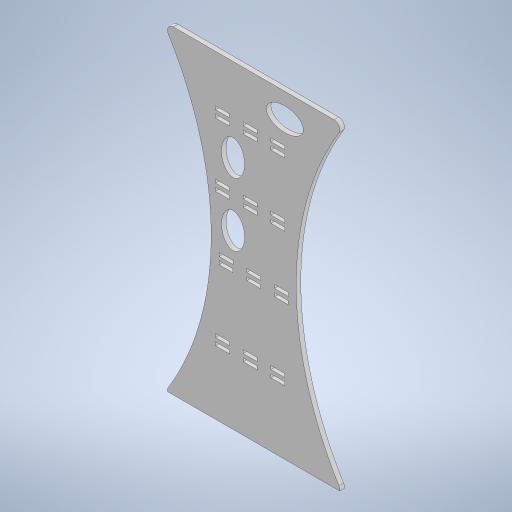
# Autodesk Inventor part: ребро
Saved by Autodesk Inventor 2023.1 (Build 271208000, 208)
## iProperties
Created: 2025-01-17
Part Number: ребро
Material: Типовые
Document SubType Name: Modeling
Designer: Коноваленко
Density: 1 g/cm^3
Appearance: По умолчанию
Author: Коноваленко
Autodesk Inventor part; units mm, degrees
ref_plane "YZ Plane" through (0, 0, 0) normal (1, 0, 0) x (0, 1, 0)
ref_plane "XZ Plane" through (0, 0, 0) normal (0, 1, 0) x (-1, 0, 0)
ref_plane "XY Plane" through (0, 0, 0) normal (0, 0, 1) x (1, 0, 0)
sketch "Эскиз1" plane through (0, 0, 0) normal (0, 0, 1) x (1, 0, 0)
  line L0 (81.8324, 0) -> (81.8324, -4) construction
  line L1 (72.759, -4) -> (11.9953, -4)
  line L2 (11.9953, -4) -> (11.9953, 0) construction
  line L3 (11.9953, 0) -> (81.8324, 0) construction
  line L4 (-75.5314, 0) -> (7.9958, 0) construction
  line L5 (7.9958, 0) -> (7.9958, -4) construction
  line L6 (7.9958, -4) -> (-66.4579, -4)
  line L7 (-75.5314, -4) -> (-75.5314, 0) construction
  line L8 (7.9953, 276) -> (11.9953, 276) construction
  line L9 (-75.5314, 0) -> (81.8324, 0)
  line L10 (72.759, 276) -> (-66.4579, 276)
  arc A0 (-70.7311, 3.5962) -> (-70.7311, 268.4038) centre (-288.6628, 136) ccw
  line L11 (3.1505, 276) -> (3.1505, 0) construction
  arc A1 (77.0322, 268.4038) -> (77.0322, 3.5962) centre (294.9639, 136) ccw
  arc A2 (-66.4579, 276) -> (-70.7311, 268.4038) centre (-66.4579, 271) ccw
  arc A3 (77.0322, 268.4038) -> (72.759, 276) centre (72.759, 271) ccw
  arc A4 (-70.7311, 3.5962) -> (-66.4579, -4) centre (-66.4579, 1) ccw
  arc A5 (72.759, -4) -> (77.0322, 3.5962) centre (72.759, 1) ccw
  point P0 (81.8324, 276)
  point P1 (-75.5314, 276)
  point P2 (-71.3569, 0)
  point P3 (77.658, 0)
  dimension "d0" = 255
  dimension "d1" = 5
  constraints: 24 end point, 16 point on circle, 8 tangent, 6 centre point, 4 point on line, 3 equal radius, 2 midpoint, 1 horizontal, 1 parallel, 1 symmetric about line, 1 other
  measures "d0" radius of A0
  measures "d1" radius of A2
extrude "Выдавливание1" add sketch "Эскиз1" along normal blind 4
sketch "Эскиз2" plane through (0, 0, 4) normal (0, 0, 1) x (1, 0, 0)
  line L0 (-29.8867, 58.1406) -> (-17.8867, 58.1406)
  line L1 (42.1133, 58.1406) -> (42.1133, 55.1406) construction
  line L2 (42.1133, 55.1406) -> (30.1133, 55.1406)
  line L3 (-29.8867, 55.1406) -> (-29.8867, 58.1406)
  line L4 (6.1133, 55.1406) -> (6.1133, 58.1406)
  line L5 (6.1133, 55.1406) -> (6.1133, 58.1406) construction
  line L6 (-17.8867, 55.1406) -> (-17.8867, 58.1406)
  line L7 (-5.8867, 55.1406) -> (-5.8867, 58.1406)
  line L8 (18.1133, 55.1406) -> (18.1133, 58.1406)
  line L9 (30.1133, 55.1406) -> (30.1133, 58.1406)
  line L10 (-17.8867, 55.1406) -> (-29.8867, 55.1406)
  line L11 (-17.8867, 58.1406) -> (-5.8867, 58.1406) construction
  line L12 (-5.8867, 58.1406) -> (6.1133, 58.1406)
  line L13 (-5.8867, 55.1406) -> (-17.8867, 55.1406) construction
  line L14 (6.1133, 58.1406) -> (18.1133, 58.1406) construction
  line L15 (18.1133, 55.1406) -> (6.1133, 55.1406) construction
  line L16 (18.1133, 58.1406) -> (30.1133, 58.1406)
  line L17 (30.1133, 58.1406) -> (42.1133, 58.1406) construction
  line L18 (30.1133, 55.1406) -> (18.1133, 55.1406)
  line L19 (6.1133, 55.1406) -> (-5.8867, 55.1406)
  line L20 (6.1133, 6.1846) -> (6.1133, 61.3406) construction
  line L21 (-29.8867, 64.3406) -> (-17.8867, 64.3406)
  line L22 (42.1133, 64.3406) -> (42.1133, 61.3406) construction
  line L23 (42.1133, 61.3406) -> (30.1133, 61.3406) construction
  line L24 (-29.8867, 61.3406) -> (-29.8867, 64.3406)
  line L25 (6.1133, 61.3406) -> (6.1133, 64.3406)
  line L26 (6.1133, 61.3406) -> (6.1133, 64.3406) construction
  line L27 (-17.8867, 61.3406) -> (-17.8867, 64.3406)
  line L28 (-5.8867, 61.3406) -> (-5.8867, 64.3406)
  line L29 (18.1133, 61.3406) -> (18.1133, 64.3406)
  line L30 (30.1133, 61.3406) -> (30.1133, 64.3406)
  line L31 (-17.8867, 61.3406) -> (-29.8867, 61.3406)
  line L32 (-17.8867, 64.3406) -> (-5.8867, 64.3406) construction
  line L33 (-5.8867, 64.3406) -> (6.1133, 64.3406)
  line L34 (-5.8867, 61.3406) -> (-17.8867, 61.3406) construction
  line L35 (6.1133, 64.3406) -> (18.1133, 64.3406) construction
  line L36 (18.1133, 61.3406) -> (6.1133, 61.3406) construction
  line L37 (18.1133, 64.3406) -> (30.1133, 64.3406)
  line L38 (30.1133, 64.3406) -> (42.1133, 64.3406) construction
  line L39 (30.1133, 61.3406) -> (18.1133, 61.3406)
  line L40 (6.1133, 61.3406) -> (-5.8867, 61.3406)
  line L41 (6.1133, -16.2034) -> (6.1133, 259.7966) construction
  line L42 (72.759, 276) -> (-66.4579, 276) projected
  line L43 (9.151, 117.4867) -> (9.151, 120.4867)
  line L44 (9.151, 117.4867) -> (9.151, 120.4867) construction
  line L45 (-2.8492, 120.4867) -> (9.151, 120.4867)
  line L46 (9.151, 117.4867) -> (-2.8492, 117.4867)
  line L47 (-2.8492, 117.4867) -> (-2.8492, 120.4867)
  line L48 (-14.8492, 117.4867) -> (-14.8492, 120.4867)
  line L49 (-14.8492, 120.4867) -> (-2.8492, 120.4867) construction
  line L50 (-2.8492, 117.4867) -> (-14.8492, 117.4867) construction
  line L51 (9.151, 62.3307) -> (9.151, 117.4867) construction
  line L52 (21.151, 117.4867) -> (9.151, 117.4867) construction
  line L53 (9.151, 120.4867) -> (21.151, 120.4867) construction
  line L54 (21.151, 117.4867) -> (21.151, 120.4867)
  line L55 (33.151, 117.4867) -> (21.151, 117.4867)
  line L56 (21.151, 120.4867) -> (33.151, 120.4867)
  line L57 (33.151, 117.4867) -> (33.151, 120.4867)
  line L58 (45.1508, 120.4867) -> (45.1508, 117.4867) construction
  line L59 (33.151, 120.4867) -> (45.1508, 120.4867) construction
  line L60 (-26.8492, 120.4867) -> (-14.8492, 120.4867)
  line L61 (-26.8492, 117.4867) -> (-26.8492, 120.4867)
  line L62 (-14.8492, 117.4867) -> (-26.8492, 117.4867)
  line L63 (-14.7362, 123.6846) -> (-14.7362, 126.6846)
  line L64 (-26.7362, 126.6846) -> (-14.7362, 126.6846)
  line L65 (-14.7362, 123.6846) -> (-26.7362, 123.6846)
  line L66 (21.2638, 123.6846) -> (21.2638, 126.6846)
  line L67 (21.2638, 126.6846) -> (33.2638, 126.6846)
  line L68 (33.2638, 123.6846) -> (33.2638, 126.6846)
  line L69 (33.2638, 123.6846) -> (21.2638, 123.6846)
  line L70 (45.2638, 126.6846) -> (45.2638, 123.6846) construction
  line L71 (21.2638, 123.6846) -> (9.2638, 123.6846) construction
  line L72 (9.2638, 126.6846) -> (21.2638, 126.6846) construction
  line L73 (9.2638, 123.6846) -> (9.2638, 126.6846)
  line L74 (9.2638, 123.6846) -> (9.2638, 126.6846) construction
  line L75 (-26.7362, 123.6846) -> (-26.7362, 126.6846)
  line L76 (33.2638, 126.6846) -> (45.2638, 126.6846) construction
  line L77 (-14.7362, 126.6846) -> (-2.7362, 126.6846) construction
  line L78 (-2.7362, 123.6846) -> (-2.7362, 126.6846)
  line L79 (-2.7362, 126.6846) -> (9.2638, 126.6846)
  line L80 (9.2638, 123.6846) -> (-2.7362, 123.6846)
  line L81 (-2.7362, 123.6846) -> (-14.7362, 123.6846) construction
  line L82 (45.2638, 123.6846) -> (33.2638, 123.6846) construction
  line L83 (6.1133, 170.9846) -> (6.1133, 173.9846)
  line L84 (6.1133, 170.9846) -> (6.1133, 173.9846) construction
  line L85 (-5.8867, 173.9846) -> (6.1133, 173.9846)
  line L86 (6.1133, 170.9846) -> (-5.8867, 170.9846)
  line L87 (-5.8867, 170.9846) -> (-5.8867, 173.9846)
  line L88 (-17.8867, 170.9846) -> (-17.8867, 173.9846)
  line L89 (-17.8867, 173.9846) -> (-5.8867, 173.9846) construction
  line L90 (-5.8867, 170.9846) -> (-17.8867, 170.9846) construction
  line L91 (18.1133, 170.9846) -> (6.1133, 170.9846) construction
  line L92 (6.1133, 173.9846) -> (18.1133, 173.9846) construction
  line L93 (18.1133, 170.9846) -> (18.1133, 173.9846)
  line L94 (30.1133, 170.9846) -> (18.1133, 170.9846)
  line L95 (18.1133, 173.9846) -> (30.1133, 173.9846)
  line L96 (30.1133, 170.9846) -> (30.1133, 173.9846)
  line L97 (42.1133, 170.9846) -> (30.1133, 170.9846) construction
  line L98 (42.1133, 173.9846) -> (42.1133, 170.9846) construction
  line L99 (30.1133, 173.9846) -> (42.1133, 173.9846) construction
  line L100 (-29.8867, 173.9846) -> (-17.8867, 173.9846)
  line L101 (-29.8867, 170.9846) -> (-29.8867, 173.9846)
  line L102 (-17.8867, 170.9846) -> (-29.8867, 170.9846)
  line L103 (6.1133, 180.1846) -> (18.1133, 180.1846) construction
  line L104 (18.1133, 177.1846) -> (6.1133, 177.1846) construction
  line L105 (18.1133, 177.1846) -> (18.1133, 180.1846)
  line L106 (30.1133, 177.1846) -> (18.1133, 177.1846)
  line L107 (18.1133, 180.1846) -> (30.1133, 180.1846)
  line L108 (-29.8867, 180.1846) -> (-17.8867, 180.1846)
  line L109 (-17.8867, 177.1846) -> (-29.8867, 177.1846)
  line L110 (-29.8867, 177.1846) -> (-29.8867, 180.1846)
  line L111 (-17.8867, 177.1846) -> (-17.8867, 180.1846)
  line L112 (30.1133, 177.1846) -> (30.1133, 180.1846)
  line L113 (42.1133, 177.1846) -> (30.1133, 177.1846) construction
  line L114 (42.1133, 180.1846) -> (42.1133, 177.1846) construction
  line L115 (30.1133, 180.1846) -> (42.1133, 180.1846) construction
  line L116 (-5.8867, 177.1846) -> (-17.8867, 177.1846) construction
  line L117 (-17.8867, 180.1846) -> (-5.8867, 180.1846) construction
  line L118 (-5.8867, 177.1846) -> (-5.8867, 180.1846)
  line L119 (6.1133, 177.1846) -> (-5.8867, 177.1846)
  line L120 (-5.8867, 180.1846) -> (6.1133, 180.1846)
  line L121 (6.1133, 177.1846) -> (6.1133, 180.1846)
  line L122 (6.1133, 177.1846) -> (6.1133, 180.1846) construction
  line L123 (6.1133, 228.9846) -> (18.1133, 228.9846) construction
  line L124 (18.1133, 225.9846) -> (6.1133, 225.9846) construction
  line L125 (18.1133, 225.9846) -> (18.1133, 228.9846)
  line L126 (30.1133, 225.9846) -> (18.1133, 225.9846)
  line L127 (18.1133, 228.9846) -> (30.1133, 228.9846)
  line L128 (-29.8867, 228.9846) -> (-17.8867, 228.9846)
  line L129 (-17.8867, 225.9846) -> (-29.8867, 225.9846)
  line L130 (-29.8867, 225.9846) -> (-29.8867, 228.9846)
  line L131 (-17.8867, 225.9846) -> (-17.8867, 228.9846)
  line L132 (30.1133, 225.9846) -> (30.1133, 228.9846)
  line L133 (42.1133, 225.9846) -> (30.1133, 225.9846) construction
  line L134 (42.1133, 228.9846) -> (42.1133, 225.9846) construction
  line L135 (30.1133, 228.9846) -> (42.1133, 228.9846) construction
  line L136 (-5.8867, 225.9846) -> (-17.8867, 225.9846) construction
  line L137 (-17.8867, 228.9846) -> (-5.8867, 228.9846) construction
  line L138 (-5.8867, 225.9846) -> (-5.8867, 228.9846)
  line L139 (6.1133, 225.9846) -> (-5.8867, 225.9846)
  line L140 (-5.8867, 228.9846) -> (6.1133, 228.9846)
  line L141 (6.1133, 225.9846) -> (6.1133, 228.9846)
  line L142 (6.1133, 225.9846) -> (6.1133, 228.9846) construction
  line L143 (18.1133, 232.1846) -> (18.1133, 235.1846)
  line L144 (30.1133, 232.1846) -> (18.1133, 232.1846)
  line L145 (18.1133, 235.1846) -> (30.1133, 235.1846)
  line L146 (30.1133, 232.1846) -> (30.1133, 235.1846)
  line L147 (42.1133, 232.1846) -> (30.1133, 232.1846) construction
  line L148 (30.1133, 235.1846) -> (42.1133, 235.1846) construction
  line L149 (42.1133, 235.1846) -> (42.1133, 232.1846) construction
  line L150 (18.1133, 232.1846) -> (6.1133, 232.1846) construction
  line L151 (6.1133, 235.1846) -> (18.1133, 235.1846) construction
  line L152 (6.1133, 232.1846) -> (6.1133, 235.1846)
  line L153 (6.1133, 232.1846) -> (6.1133, 235.1846) construction
  line L154 (6.1133, 232.1846) -> (-5.8867, 232.1846)
  line L155 (-5.8867, 235.1846) -> (6.1133, 235.1846)
  line L156 (-5.8867, 232.1846) -> (-5.8867, 235.1846)
  line L157 (-5.8867, 232.1846) -> (-17.8867, 232.1846) construction
  line L158 (-17.8867, 235.1846) -> (-5.8867, 235.1846) construction
  line L159 (-17.8867, 232.1846) -> (-17.8867, 235.1846)
  line L160 (-29.8867, 235.1846) -> (-17.8867, 235.1846)
  line L161 (-29.8867, 232.1846) -> (-29.8867, 235.1846)
  line L162 (-17.8867, 232.1846) -> (-29.8867, 232.1846)
  arc A0 (-70.7311, 3.5962) -> (-70.7311, 268.4038) centre (-288.6628, 136) ccw construction
  arc A1 (77.0322, 268.4038) -> (77.0322, 3.5962) centre (294.9639, 136) ccw construction
  line L163 (-26.8492, 117.4867) -> (-34.3357, 117.4867)
  line L164 (33.151, 117.4867) -> (40.6375, 117.4765)
  point P0 (0, 0)
  point P1 (-29.8867, 56.6406)
  point P2 (-17.8867, 56.6406)
  point P3 (-5.8867, 56.6406)
  point P4 (6.1133, 56.6406)
  point P5 (18.1133, 56.6406)
  point P6 (30.1133, 56.6406)
  point P7 (6.1133, 62.8406)
  point P8 (-29.8867, 62.8406)
  point P9 (-17.8867, 62.8406)
  point P10 (-5.8867, 62.8406)
  point P11 (6.1133, 62.8406)
  point P12 (18.1133, 62.8406)
  point P13 (30.1133, 62.8406)
  point P14 (6.1133, 117.4846)
  point P15 (9.2638, 118.9846)
  point P16 (9.151, 118.9867)
  point P17 (-2.8492, 118.9867)
  point P18 (21.151, 118.9867)
  point P19 (33.151, 118.9867)
  point P20 (-14.8492, 118.9867)
  point P21 (-26.8492, 118.9867)
  point P22 (6.1133, 123.6846)
  point P23 (6.1133, 123.6846)
  point P24 (21.2638, 125.1846)
  point P25 (33.2638, 125.1846)
  point P26 (9.2638, 125.1846)
  point P27 (-26.7362, 125.1846)
  point P28 (-2.7362, 125.1846)
  point P29 (-14.7362, 125.1846)
  point P30 (9.2638, 125.1846)
  point P31 (6.1133, 170.9846)
  point P32 (3.2638, 126.6846)
  point P33 (30.1133, 172.4846)
  point P34 (-17.8867, 172.4846)
  point P35 (-29.8867, 172.4846)
  point P36 (6.1133, 177.1846)
  point P37 (-17.8867, 178.6846)
  point P38 (-29.8867, 178.6846)
  point P39 (30.1133, 178.6846)
  point P40 (6.1133, 178.6846)
  point P41 (6.1133, 225.9846)
  point P42 (6.1133, 225.9846)
  point P43 (18.1133, 227.4846)
  point P44 (-17.8867, 227.4846)
  point P45 (-29.8867, 227.4846)
  point P46 (30.1133, 227.4846)
  point P47 (-5.8867, 227.4846)
  point P48 (18.1133, 233.6846)
  point P49 (30.1133, 233.6846)
  point P50 (-5.8867, 233.6846)
  point P51 (-17.8867, 233.6846)
  point P52 (-29.8867, 233.6846)
  point P53 (6.1133, 232.1846)
  point P54 (6.1133, 225.9846)
  point P55 (0.1133, 180.1846)
  dimension "d15" = 72
  dimension "d16" = 3
  dimension "d18" = 12
  dimension "d19" = 12
  dimension "d20" = 12
  dimension "d21" = 12
  dimension "d22" = 4.7
  dimension "d23" = 72
  dimension "d24" = 3
  dimension "d25" = 12
  dimension "d26" = 12
  dimension "d27" = 12
  dimension "d28" = 12
  dimension "d37" = 72
  dimension "d38" = 3
  dimension "d39" = 12
  dimension "d40" = 12
  dimension "d41" = 12
  dimension "d42" = 12
  dimension "d44" = 72
  dimension "d45" = 3
  dimension "d46" = 12
  dimension "d47" = 12
  dimension "d48" = 12
  dimension "d49" = 12
  dimension "d51" = 44.3
  dimension "d52" = 72
  dimension "d53" = 3
  dimension "d54" = 12
  dimension "d59" = 72
  dimension "d60" = 3
  dimension "d61" = 12
  dimension "d66" = 72
  dimension "d67" = 3
  dimension "d68" = 12
  dimension "d69" = 12
  dimension "d71" = 12
  dimension "d73" = 72
  dimension "d74" = 3
  dimension "d75" = 12
  dimension "d76" = 12
  dimension "d78" = 12
  dimension "d79" = 45.8
  constraints: 328 end point, 290 parallel, 239 perpendicular, 88 point on line, 49 horizontal, 43 midpoint, 11 vertical, 2 point on circle, 1 equal length
  measures "d15" distance of L1.end L3.start
  measures "d16" distance of L1.start L1.end
  measures "d18" distance of point (-29.887, 56.641) point (-17.887, 56.641)
  measures "d19" distance of point (-5.887, 56.641) point (-17.887, 56.641)
  measures "d20" distance of point (6.113, 56.641) point (18.113, 56.641)
  measures "d21" distance of point (30.113, 56.641) point (18.113, 56.641)
  measures "d22" distance from line of point (6.113, 62.841) L12
  measures "d23" distance of L23.start L24.start
  measures "d24" distance of L22.start L23.start
  measures "d25" distance of point (-29.887, 62.841) point (-17.887, 62.841)
  measures "d26" distance of point (-5.887, 62.841) point (-17.887, 62.841)
  measures "d27" distance of point (6.113, 62.841) point (18.113, 62.841)
  measures "d28" distance of point (30.113, 62.841) point (18.113, 62.841)
  measures "d37" distance of L58.end L62.end
  measures "d38" distance of L58.start L58.end
  measures "d39" distance of point (-26.849, 118.987) point (-14.849, 118.987)
  measures "d40" distance of point (-2.849, 118.987) point (-14.849, 118.987)
  measures "d41" distance of point (9.151, 118.987) point (21.151, 118.987)
  measures "d42" distance of point (33.151, 118.987) point (21.151, 118.987)
  measures "d44" distance of L82.start L65.end
  measures "d45" distance of L76.end L82.start
  measures "d46" distance of point (-26.736, 125.185) point (-14.736, 125.185)
  measures "d47" distance of point (-2.736, 125.185) point (-14.736, 125.185)
  measures "d48" distance of point (9.264, 125.185) point (21.264, 125.185)
  measures "d49" distance of point (33.264, 125.185) point (21.264, 125.185)
  measures "d51" vertical distance of point (3.264, 126.685) point (6.113, 170.985)
  measures "d52" distance of L97.start L102.end
  measures "d53" distance of L98.start L97.start
  measures "d54" distance of point (-29.887, 172.485) point (-17.887, 172.485)
  measures "d59" distance of L113.start L110.start
  measures "d60" distance of L115.end L113.start
  measures "d61" distance of point (-29.887, 178.685) point (-17.887, 178.685)
  measures "d66" distance of L133.start L129.end
  measures "d67" distance of L134.start L133.start
  measures "d68" distance of point (-29.887, 227.485) point (-17.887, 227.485)
  measures "d69" distance of point (-5.887, 227.485) point (-17.887, 227.485)
  measures "d71" distance of point (30.113, 227.485) point (18.113, 227.485)
  measures "d73" distance of L147.start L162.end
  measures "d74" distance of L148.end L147.start
  measures "d75" distance of point (-29.887, 233.685) point (-17.887, 233.685)
  measures "d76" distance of point (-5.887, 233.685) point (-17.887, 233.685)
  measures "d78" distance of point (30.113, 233.685) point (18.113, 233.685)
  measures "d79" vertical distance of point (6.113, 225.985) point (0.113, 180.185)
extrude "Выдавливание2" cut sketch "Эскиз2" against normal blind 10
sketch "Эскиз3" plane through (0, 0, 0) normal (0, 0, -1) x (-1, 0, 0)
  line L0 (29.8867, 235.1846) -> (29.8867, 232.1846)
  line L1 (5.8867, 232.1846) -> (5.8867, 235.1846) construction
  line L2 (29.8867, 235.1846) -> (17.8867, 235.1846) construction
  line L3 (5.8867, 235.1846) -> (17.8867, 235.1846) construction
  line L4 (17.8867, 235.1846) -> (17.8867, 282.8857) construction
  line L5 (-72.759, 276) -> (66.4579, 276) construction
  line L6 (-72.759, 276) -> (66.4579, 276) projected
  line L7 (-3.1505, 276) -> (-3.1505, 0) construction
  ellipse E0 centre (14.7362, 203.914) end of major axis (14.7362, 188.914) minor radius 10
  ellipse E1 centre (14.7362, 149.1217) end of major axis (14.7362, 134.1217) minor radius 10
  line L8 (26.9627, 126.6846) -> (14.9627, 126.6846) construction
  line L9 (14.9627, 126.6846) -> (26.9627, 126.6846)
  ellipse E2 centre (-30.1133, 255.0594) end of major axis (-46.1133, 255.0594) minor radius 10
  line L10 (-30.1133, 232.1846) -> (-30.1133, 235.1846) projected
  line L11 (-18.1133, 235.1846) -> (-30.1133, 235.1846) projected
  line L12 (-30.1133, 235.1846) -> (-30.1133, 279.5506) construction
  line L13 (26.7362, 126.6846) -> (14.7362, 126.6846) projected
  line L14 (14.7362, 126.6846) -> (14.7362, 287.1636) construction
  line L15 (14.7362, 126.6846) -> (175.2152, 126.6846) construction
  point P0 (0, 0)
  point P1 (-33.2638, 126.6846)
  point P2 (-21.2638, 126.6846)
  dimension "d92" = 16
  dimension "d90" = 160.479
  dimension "d91" = 90
  constraints: 18 end point, 3 perpendicular, 3 point on line, 2 centre point, 2 horizontal, 2 symmetric about line, 2 vertical, 1 midpoint, 2 other
  measures "d90" distance of L13.end L14.end
  measures "d91" angle of L15 L14
extrude "Выдавливание3" cut sketch "Эскиз3" against normal blind 10
